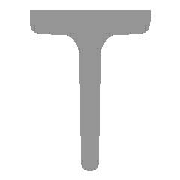
# Autodesk Inventor part: DIN 1024 - T30-900
Saved by Autodesk Inventor 2018 (Build 220112000, 112)
## iProperties
IsCustomPart: 1
_CCFamilyMember: 30
_CCFamilyDisplayName: DIN 1024 - Hot rolled T-bars — DIN 1024 was withdrawn and replaced by DIN EN 10055
_FrameMemberDoc: Frame Member File
_Version: 15.0.0
_GetPNFromCC: 1
Created: 2017-02-09
Part Number: DIN 1024 - T30-900
Material: Steel, Mild
Description: Hot rolled T-bars
Document SubType Name: Modeling
Standard: DIN
Designer: gust3763
Standards Organization: DIN
Language: en-US
Size Designation: T30
Categories: <MemberInstance><Categories><Category DisplayName="Structural Shapes" InternalName="089c4875-fa83-4c05-b084-43b9cc11f5ed" Mnemonic="GRDR"><CategoryParameter DisplayName="Mass per Length Unit" InternalName="0bb95a10-148f-4027-a459-38d7b056702a" Mnemonic="shpmass"/><CategoryParameter DisplayName="Section Area" InternalName="1ff91680-64b0-4202-b9a3-7fd3f94bba3b" Mnemonic="secarea"/><CategoryParameter DisplayName="Radius of Gyration (x)" InternalName="25778675-03e9-40c1-b6a8-4a9ed693320d" Mnemonic="gyrradx"/><CategoryParameter DisplayName="Torsional Rigidity Modulus" InternalName="26c1ec35-5026-4c63-ad0a-751cf684a536" Mnemonic="torrigmod"/><CategoryParameter DisplayName="Distance of the Center of Gravity X-X" InternalName="26c9bdb8-9c79-4b4f-a92e-8e197583c9c4" Mnemonic="grcendistX"/><CategoryParameter DisplayName="Legacy Member ID" InternalName="340afe4f-75d7-48d3-ab7d-943f3c3da468" Mnemonic="LegacyMemberID"/><CategoryParameter DisplayName="Base Length" InternalName="42e34263-8f20-4d0e-ad48-bf1385b87c24" Mnemonic="shplen"/><CategoryParameter DisplayName="Moment of Inertia (y)" InternalName="4b9f58ea-bced-460e-81ea-3d29ca5a49e3" Mnemonic="inermomy"/><CategoryParameter DisplayName="Moment of Inertia (x)" InternalName="4cd780bc-73d7-43ac-917a-579e5cbd684d" Mnemonic="inermomx"/><CategoryParameter DisplayName="Custom Base Point" InternalName="4f1d1b73-316d-484b-a3df-9cbabb16eb77" Mnemonic="shpBasePoint"/><CategoryParameter DisplayName="Shape Height" InternalName="50274e7d-5ac0-4796-92cb-c59e54983c67" Mnemonic="shpheig"/><CategoryParameter DisplayName="Section Module (y)" InternalName="59eaa5e9-d227-48dc-b6c1-6920f96e0f95" Mnemonic="secmody"/><CategoryParameter DisplayName="Section Designation" InternalName="5a64d034-428d-49c8-ba32-7619764de20f" Mnemonic="shpdes"/><CategoryParameter DisplayName="Section Module (x)" InternalName="72cfad18-cf51-4ed4-aaa7-c6b224f8419f" Mnemonic="secmodx"/><CategoryParameter DisplayName="Torsional Section Modulus" InternalName="7c55a8dc-8844-49f9-a867-cc677b30ec9a" Mnemonic="torsecmod"/><CategoryParameter DisplayName="Shape Width" InternalName="7c717d54-a18f-4666-b4d4-573cce22c62c" Mnemonic="shpwdth"/><CategoryParameter DisplayName="Second Shape Thickness" InternalName="9251a8e1-85fd-4e47-af99-afdb762317d9" Mnemonic="shpthick2"/><CategoryParameter DisplayName="FG Authored" InternalName="9c666724-f362-4ea7-ac62-f6a007de5c69" Mnemonic="shpFGAuto"/><CategoryParameter DisplayName="Distance of the Center of Gravity Y-Y" InternalName="bcc4fb17-7af4-436a-8f8c-d0aa3b0248c5" Mnemonic="grcendistY"/><CategoryParameter DisplayName="Radius of Gyration (y)" InternalName="bfa18ebe-1636-4dbe-8d42-b263e0b73184" Mnemonic="gyrrady"/><CategoryParameter DisplayName="Shape Thickness" InternalName="d109cf76-8eb4-42fc-9800-4409734adc67" Mnemonic="shpthick"/><CategoryParameter DisplayName="Coefficient of Shear Displacement" InternalName="de4c90c6-aaa8-468f-a335-6737b311b5d3" Mnemonic="shdispc"/><Category DisplayName="Tees" InternalName="56b6ab2f-f472-4170-92b4-e80ee6bbd321" Mnemonic="TSHP"><CategoryParameter DisplayName="Second Shape Thickness" InternalName="0c030a53-361c-42d0-87b6-901a5d97f52b" Mnemonic="shpthick2"/><CategoryParameter DisplayName="Moment of Inertia (y)" InternalName="166217f1-0ffb-49df-8876-ca0594e212d8" Mnemonic="inermomy"/><CategoryParameter DisplayName="Shape Thickness" InternalName="4e82dedf-7d13-47ae-bb3d-701facb8d0f8" Mnemonic="shpthick"/><CategoryParameter DisplayName="Section Area" InternalName="62f9067b-d4e2-4bd7-90dd-bf9a2a8725dd" Mnemonic="secarea"/><CategoryParameter DisplayName="Radius of Gyration (x)" InternalName="9a0e3113-fceb-4297-9bb9-aaf636d26195" Mnemonic="gyrradx"/><CategoryParameter DisplayName="Section Module (x)" InternalName="a2b125e9-258c-48f9-8bec-bf10c8c20659" Mnemonic="secmodx"/><CategoryParameter DisplayName="Shape Width" InternalName="dfb96244-4609-45f3-9c9f-349c0965565b" Mnemonic="shpwdth"/><CategoryParameter DisplayName="Section Module (y)" InternalName="e74eb2df-3e61-41c9-8373-664904bb7552" Mnemonic="secmody"/><CategoryParameter DisplayName="Radius of Gyration (y)" InternalName="f8f84113-8c08-48b5-bbf8-282dee0d2626" Mnemonic="gyrrady"/><CategoryParameter DisplayName="Moment of Inertia (x)" InternalName="fe31bfef-9845-423b-866e-9b8501e64c72" Mnemonic="inermomx"/></Category></Category><Category DisplayName="DataType" InternalName="23b78d0f-2648-40c6-8793-ca6db495c9e8" Mnemonic="DATATYPE"><CategoryParameter DisplayName="DisplayName" InternalName="05415f3d-3907-474b-a020-eb9d644f4cf3" Mnemonic="DISPLAYNAME"/><CategoryParameter DisplayName="Standard" InternalName="0c0a119c-1e12-4c84-803f-101930972f5e" Mnemonic="STANDARD"/><CategoryParameter DisplayName="Description" InternalName="13903e3d-64b1-4950-80da-f627842ea37f" Mnemonic="DESCRIPTION"/><CategoryParameter DisplayName="Designation" InternalName="2675968c-4ce5-49e0-a4f5-552d29089031" Mnemonic="DESIGNATION"/><CategoryParameter DisplayName="Default Row" InternalName="2af9ec52-faaa-4026-b378-f9fa4afca842" Mnemonic="DEFAULTROW"/><CategoryParameter DisplayName="Folder Name" InternalName="3f06958e-8713-4116-9be7-ed6184ecc97b" Mnemonic="FOLDERNAME"/><CategoryParameter DisplayName="Revision Guid" InternalName="45a75005-10b1-4dfc-8d6d-dfe629f0b93c" Mnemonic="REVISIONGUID"/><CategoryParameter DisplayName="FileName" InternalName="8b46a4cc-9585-4fed-90c3-899f57e09a73" Mnemonic="FILENAME"/><CategoryParameter DisplayName="StdsOrg" InternalName="8f5914e1-4693-403f-8ab5-d37768198c9d" Mnemonic="STDSORG"/><CategoryParameter DisplayName="Family Version" InternalName="914462f6-6e19-4b14-ba84-155b9680b1d0" Mnemonic="FAMILYREVISION"/><CategoryParameter DisplayName="Standard Revision" InternalName="91d5a463-65c2-4fde-b823-3b7fea5e8e17" Mnemonic="STANDARDREVISION"/><CategoryParameter DisplayName="Member Revision" InternalName="a65d44b9-392f-4f4f-857b-e4b3d54996fe" Mnemonic="MEMBERREVISION"/><CategoryParameter DisplayName="ClipFormat" InternalName="bc51e27b-3422-4e78-93ef-cec197ddf230" Mnemonic="CLIPFORMAT"/><CategoryParameter DisplayName="Manufacturer" InternalName="cd6c7a72-a28a-4e50-99a9-2c7f4e13e5ad" Mnemonic="MANUFACTURER"/><CategoryParameter DisplayName="InternalName" InternalName="cf1d0246-76d9-4b4a-8305-fa0409afb5c1" Mnemonic="INTERNALNAME"/><CategoryParameter DisplayName="IsMetric" InternalName="e2385c5b-1ea4-4823-96a8-8de651266ec3" Mnemonic="ISMETRIC"/><Category DisplayName="Part" InternalName="c0e0b642-3bcb-4cc8-9e80-f96d35c4afa4" Mnemonic="PART"><CategoryParameter DisplayName="Part Number" InternalName="016b6077-bfbe-49bd-92c9-d8d59c39c941" Mnemonic="PARTNUMBER"/><CategoryParameter DisplayName="Stock Number" InternalName="4dba7c1c-e26c-444e-836c-b08b433409a8" Mnemonic="STOCKNUMBER"/><CategoryParameter DisplayName="Material Key" InternalName="5c9a8adb-dd2b-4535-b97f-0a94a95fe41f" Mnemonic="MATERIALKEY"/><CategoryParameter DisplayName="Material" InternalName="818a152a-d3c3-49ca-80ee-df7d91421b8e" Mnemonic="MATERIAL"/></Category></Category><Category DisplayName="Legacy Map DA" InternalName="924fff40-ddd0-4eff-ad42-30e3774ef79e" Mnemonic="LEGACYMAPDA"><CategoryParameter DisplayName="DACookie" InternalName="316934ee-8fe1-4c7a-9c36-f2d79e1add1a" Mnemonic="DACOOKIE"/></Category></Categories><FamilyTemplate Id="N425580"><FamilyTemplateParameters><FamilyTemplateParameter ObjectType="kUserParameterObject" ValueType="xs:double" Id="1" ObjectReferenceKey="ParH"/><FamilyTemplateParameter ObjectType="kUserParameterObject" ValueType="xs:double" Id="2" ObjectReferenceKey="b"/><FamilyTemplateParameter ObjectType="kUserParameterObject" ValueType="xs:double" Id="3" ObjectReferenceKey="ParT"/><FamilyTemplateParameter ObjectType="kUserParameterObject" ValueType="xs:double" Id="4" ObjectReferenceKey="B_L"/><FamilyTemplateParameter ObjectType="kUserParameterObject" ValueType="xs:double" Id="5" ObjectReferenceKey="R"/><FamilyTemplateParameter ObjectType="kUserParameterObject" ValueType="xs:double" Id="6" ObjectReferenceKey="R1"/><FamilyTemplateParameter ObjectType="kUserParameterObject" ValueType="xs:double" Id="7" ObjectReferenceKey="R2"/><FamilyTemplateParameter ObjectType="kUserParameterObject" ValueType="xs:double" Id="8" ObjectReferenceKey="ex"/><FamilyTemplateParameter ObjectType="kPropertyObject" ValueType="xs:string" Id="100" ObjectReferenceKey="{32853F0F-3444-11d1-9E93-0060B03C1CA6}" SubObjectId="52"/><FamilyTemplateParameter ObjectType="kPropertyObject" ValueType="xs:string" Id="105" ObjectReferenceKey="{32853F0F-3444-11d1-9E93-0060B03C1CA6}" SubObjectId="5"/><FamilyTemplateParameter ObjectType="kPartComponentDefinitionObject" ValueType="xs:string" Id="110" SubObjectId="Material"/><FamilyTemplateParameter ObjectType="kPropertyObject" ValueType="xs:string" Id="112" ObjectReferenceKey="{32853F0F-3444-11d1-9E93-0060B03C1CA6}" SubObjectId="55"/></FamilyTemplateParameters></FamilyTemplate><CategoryParameterMap><ParamToTemplateMap><ParamToTemplate CategoryParameter="//CategoryParameter[@InternalName='05415f3d-3907-474b-a020-eb9d644f4cf3']" ConstantValue="DIN 1024"/><ParamToTemplate CategoryParameter="//CategoryParameter[@InternalName='cf1d0246-76d9-4b4a-8305-fa0409afb5c1']" ConstantValue="3BAF420C-5161-48F7-92A1-AA756BD9F78E"/><ParamToTemplate CategoryParameter="//CategoryParameter[@InternalName='3f06958e-8713-4116-9be7-ed6184ecc97b']" ConstantValue="DIN 1024"/><ParamToTemplate CategoryParameter="//CategoryParameter[@InternalName='914462f6-6e19-4b14-ba84-155b9680b1d0']" ConstantValue="10"/><ParamToTemplate CategoryParameter="//CategoryParameter[@InternalName='bc51e27b-3422-4e78-93ef-cec197ddf230']" ConstantValue="CF_INVENTOR.STDPARTS"/><ParamToTemplate CategoryParameter="//CategoryParameter[@InternalName='e2385c5b-1ea4-4823-96a8-8de651266ec3']" ConstantValue="true"/><ParamToTemplate CategoryParameter="//CategoryParameter[@InternalName='13903e3d-64b1-4950-80da-f627842ea37f']" ConstantValue="Hot rolled T-bars"/><ParamToTemplate CategoryParameter="//CategoryParameter[@InternalName='8f5914e1-4693-403f-8ab5-d37768198c9d']" ConstantValue="DIN"/><ParamToTemplate CategoryParameter="//CategoryParameter[@InternalName='0c0a119c-1e12-4c84-803f-101930972f5e']" ConstantValue="DIN 1024"/><ParamToTemplate CategoryParameter="//CategoryParameter[@InternalName='cd6c7a72-a28a-4e50-99a9-2c7f4e13e5ad']" TemplateParameter="104"/><ParamToTemplate CategoryParameter="//CategoryParameter[@InternalName='91d5a463-65c2-4fde-b823-3b7fea5e8e17']" TemplateParameter="103"/><ParamToTemplate CategoryParameter="//CategoryParameter[@InternalName='45a75005-10b1-4dfc-8d6d-dfe629f0b93c']" ConstantValue="b59734f9-a795-4362-8abe-aa75fb9b97fd"/><ParamToTemplate CategoryParameter="//CategoryParameter[@InternalName='2af9ec52-faaa-4026-b378-f9fa4afca842']" ConstantValue="10"/><ParamToTemplate CategoryParameter="//CategoryParameter[@InternalName='9c666724-f362-4ea7-ac62-f6a007de5c69']" ConstantValue="1"/><ParamToTemplate CategoryParameter="//CategoryParameter[@InternalName='8b46a4cc-9585-4fed-90c3-899f57e09a73']" ConstantValue="DIN 1024 - T30-1"/><ParamToTemplate CategoryParameter="//CategoryParameter[@InternalName='a65d44b9-392f-4f4f-857b-e4b3d54996fe']" ConstantValue="A2B3531A-96C3-4959-AD6D-F7BB062883CD"/><ParamToTemplate CategoryParameter="//CategoryParameter[@InternalName='fe31bfef-9845-423b-866e-9b8501e64c72']" ConstantValue="17200"/><ParamToTemplate CategoryParameter="//CategoryParameter[@InternalName='166217f1-0ffb-49df-8876-ca0594e212d8']" ConstantValue="8700"/><ParamToTemplate CategoryParameter="//CategoryParameter[@InternalName='a2b125e9-258c-48f9-8bec-bf10c8c20659']" ConstantValue="800"/><ParamToTemplate CategoryParameter="//CategoryParameter[@InternalName='e74eb2df-3e61-41c9-8373-664904bb7552']" ConstantValue="580"/><ParamToTemplate CategoryParameter="//CategoryParameter[@InternalName='62f9067b-d4e2-4bd7-90dd-bf9a2a8725dd']" ConstantValue="226"/><ParamToTemplate CategoryParameter="//CategoryParameter[@InternalName='7c55a8dc-8844-49f9-a867-cc677b30ec9a']" ConstantValue="331,52"/><ParamToTemplate CategoryParameter="//CategoryParameter[@InternalName='26c1ec35-5026-4c63-ad0a-751cf684a536']" ConstantValue="1326,08"/><ParamToTemplate CategoryParameter="//CategoryParameter[@InternalName='de4c90c6-aaa8-468f-a335-6737b311b5d3']" ConstantValue="2,1"/><ParamToTemplate CategoryParameter="//CategoryParameter[@InternalName='316934ee-8fe1-4c7a-9c36-f2d79e1add1a']" ConstantValue="*DIN~D1024~T30-25000*"/><ParamToTemplate CategoryParameter="//CategoryParameter[@InternalName='42e34263-8f20-4d0e-ad48-bf1385b87c24']" TemplateParameter="4"/><ParamToTemplate CategoryParameter="//CategoryParameter[@InternalName='2675968c-4ce5-49e0-a4f5-552d29089031']" TemplateParameter="100"/><ParamToTemplate CategoryParameter="//CategoryParameter[@InternalName='818a152a-d3c3-49ca-80ee-df7d91421b8e']" TemplateParameter="110"/><ParamToTemplate CategoryParameter="//CategoryParameter[@InternalName='016b6077-bfbe-49bd-92c9-d8d59c39c941']" TemplateParameter="105"/><ParamToTemplate CategoryParameter="//CategoryParameter[@InternalName='50274e7d-5ac0-4796-92cb-c59e54983c67']" TemplateParameter="1"/><ParamToTemplate CategoryParameter="//CategoryParameter[@InternalName='4dba7c1c-e26c-444e-836c-b08b433409a8']" TemplateParameter="112"/><ParamToTemplate CategoryParameter="//CategoryParameter[@InternalName='26c9bdb8-9c79-4b4f-a92e-8e197583c9c4']" TemplateParameter="8"/></ParamToTemplateMap></CategoryParameterMap></MemberInstance>
Stock Number: T30
Density: 7.85 g/cm^3
Appearance: Semi-Polished
G_L: 900,000 mm
G_W: 30,000 mm
G_H: 30,000 mm
Author: gust3763
Autodesk Inventor part; units mm, degrees
ref_plane "YZ Plane" through (0, 0, 0) normal (1, 0, 0) x (0, 1, 0)
ref_plane "WorkPlane3" through (0, 0, 0) normal (0, 1, 0) x (-1, 0, 0)
ref_plane "XY Plane" through (0, 0, 0) normal (0, 0, 1) x (1, 0, 0)
ref_plane "Start plane" through (0, 0, 0) normal (0, 0, 1) x (1, 0, 0)
ref_plane "End plane" through (0, 0, 900) normal (0, 0, 1) x (1, 0, 0)
sketch "Sketch" plane through (0, 0, 0) normal (0, 0, 1) x (1, 0, 0)
  line L0 (0.8698, -38.5) -> (-0.8698, -38.5)
  line L1 (2.2911, -16.445) -> (1.8696, -37.52)
  line L2 (13.04, -12.3892) -> (6.2103, -12.5258)
  line L3 (15, -8.5) -> (15, -10.3896)
  line L4 (-15, -10.3896) -> (-15, -8.5)
  line L5 (-6.2103, -12.5258) -> (-13.04, -12.3892)
  line L6 (-1.8696, -37.52) -> (-2.2911, -16.445)
  line L7 (-2.3679, -12.6026) -> (2.3679, -12.6026) construction
  line L8 (0, -46.445) -> (0, 7.7408) construction
  arc A0 (-2.2911, -16.445) -> (-6.2103, -12.5258) centre (-6.2903, -16.525) ccw
  arc A1 (6.2103, -12.5258) -> (2.2911, -16.445) centre (6.2903, -16.525) ccw
  arc A2 (-15, -10.3896) -> (-13.04, -12.3892) centre (-13, -10.3896) ccw
  arc A3 (13.04, -12.3892) -> (15, -10.3896) centre (13, -10.3896) ccw
  arc A4 (-1.8696, -37.52) -> (-0.8698, -38.5) centre (-0.8698, -37.5) ccw
  arc A5 (0.8698, -38.5) -> (1.8696, -37.52) centre (0.8698, -37.5) ccw
  line L9 (-21.5716, 0) -> (21.5716, 0) construction
  line L10 (-15, -8.5) -> (15, -8.5)
  point P0 (1.85, -38.5)
  point P1 (-1.85, -38.5)
  point P2 (15, -12.35)
  point P3 (-15, -12.35)
  point P4 (0, 0)
  point P5 (0, -12.6026)
  dimension "d9" = 3.85
  dimension "d11" = 3.85
  dimension "d23" = 3.7
  dimension "d26" = 1.146
  dimension "d27" = 1.146
  dimension "d28" = 4
  dimension "d29" = 2
  dimension "d30" = 1
  dimension "d31" = 30
  dimension "d32" = 1.146
  dimension "d33" = 30
  dimension "d34" = 8.5
  constraints: 18 end point, 13 point on line, 12 point on circle, 12 tangent, 6 centre point, 3 equal radius, 2 horizontal, 2 vertical, 1 equal length, 1 midpoint, 1 parallel
  measures "d9" distance of L3.start point (15, -12.35)
  measures "d11" distance of point (-15, -12.35) L4.end
  measures "d23" distance of point (1.85, -38.5) point (-1.85, -38.5)
  measures "d26" angle of L8 L1
  measures "d27" angle of L6 L8
  measures "d28" radius of A0
  measures "d29" radius of A2
  measures "d30" radius of A4
  measures "d31" distance from line of L10 point (1.85, -38.5)
  measures "d32" angle of L2 L9
  measures "d33" distance of L4.end L3.start
  measures "d34" distance between parallel lines of L9 L10
extrude "Body" add sketch "Sketch" along normal up to surface (900 mm away) from surface at 0
sketch "Sketch3" plane through (0, 0, 0) normal (0, 0, 1) x (1, 0, 0)
  line L0 (0, 0) -> (10, 0)
ref_plane "Work Plane6" through (0, 0, 0) normal (0, -1, 0) x (1, 0, 0)
sketch "Sketch4" plane through (0, 0, 0) normal (0, -1, 0) x (1, 0, 0)
  line L0 (-2, 0) -> (12, 0)
  line L1 (-2, 900) -> (12, 900)
  dimension "d38" = 900
  measures "d38" distance between parallel lines of L0 L1
equation "\"d9\" = -msp_pom3 + ParT"
equation "\"d11\" = -msp_pom3 + ParT"
equation "\"d23\" = ParT - msp_pom2"
equation "\"d26\" = d27"
equation "\"d27\" = d32"
equation "\"d28\" = R"
equation "\"d29\" = R1"
equation "\"d30\" = R2"
equation "\"d31\" = ParH"
equation "\"d32\" = msp_ang"
equation "\"d33\" = b"
equation "\"d34\" = ex"
equation "\"d13\" = G_L"
equation "\"b\" = 30"
equation "\"ParH\" = 30"
equation "\"R\" = 4"
equation "\"ParT\" = 4"
equation "\"R1\" = 2"
equation "\"R2\" = 1"
equation "\"G_L\" = d38"
equation "\"msp_x1\" = 0"
equation "\"msp_x2\" = 0"
equation "\"msp_x\" = 0"
equation "\"msp_ang\" = 1.14576deg"
equation "\"ex\" = 8.5"
equation "\"G_OFFSET_START\" = 0"
equation "\"G_OFFSET_END\" = 0"
equation "\"msp_pom3\" = 0.15"
equation "\"msp_pom2\" = 0.3"
body "Solid1"
